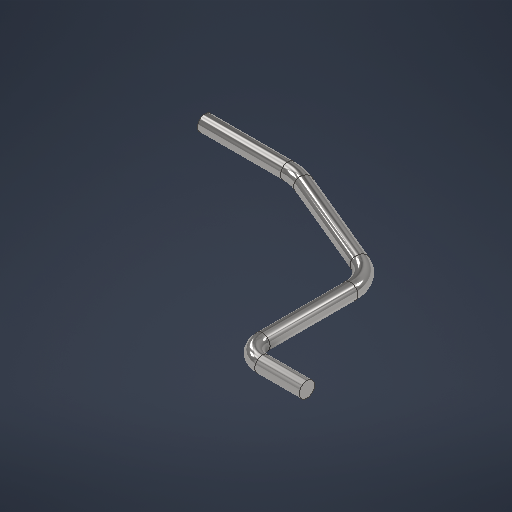
# Autodesk Inventor part: front iron bar
Saved by Autodesk Inventor 2026.1 (Build 301233000, 233)
## iProperties
Created: 2025-12-10
Part Number: front iron bar
Material: Generisch
Document SubType Name: Modeling
Designer: Familie
Density: 1 g/cm^3
Appearance: Stahl - poliert
Author: Familie
Autodesk Inventor part; units mm, degrees
ref_plane "YZ Plane" through (0, 0, 0) normal (1, 0, 0) x (0, 1, 0)
ref_plane "XZ Plane" through (0, 0, 0) normal (0, 1, 0) x (-1, 0, 0)
ref_plane "XY Plane" through (0, 0, 0) normal (0, 0, 1) x (1, 0, 0)
sketch "Skizze1" plane through (0, 0, 0) normal (0, 0, 1) x (1, 0, 0)
  line L0 (0, 0) -> (15, 0)
  arc A0 (20, -1) -> (15, 0) centre (15, -13) ccw
  line L1 (20, -1) -> (45, -11.4167)
  arc A1 (50, -18.9167) -> (45, -11.4167) centre (41.875, -18.9167) ccw
  line L2 (50, -18.9167) -> (50, -41.6467)
  arc A2 (50, -41.6467) -> (55, -46.6467) centre (55, -41.6467) ccw
  line L3 (55, -46.6467) -> (60, -46.6467)
  line L4 (60, -46.6467) -> (66.5, -46.6467)
  line L5 (0, 0) -> (-6.5, 0)
  point P0 (57.5, -46.6467)
  dimension "d0" = 15
  dimension "d1" = 20
  dimension "d2" = 1
  dimension "d3" = 45
  dimension "d4" = 5
  dimension "d5" = 22.73
  dimension "d6" = 5
  dimension "d7" = 5
  dimension "d20" = 46.6467
  dimension "d22" = 6.5
  dimension "d23" = 6.5
  constraints: 12 end point, 6 point on circle, 6 tangent, 4 horizontal, 3 centre point, 1 midpoint, 1 vertical
  measures "d0" distance of L0.start L0.end
  measures "d1" horizontal distance of L1.start L0.start
  measures "d2" vertical distance of L0.end L1.start
  measures "d3" horizontal distance of L0.start L1.end
  measures "d4" horizontal distance of L1.end L2.start
  measures "d5" distance of L2.start L2.end
  measures "d6" horizontal distance of L2.end L3.start
  measures "d7" distance of L3.start L3.end
  measures "d20" distance between parallel lines of L3 L0
  measures "d22" distance of L3.end L4.end
  measures "d23" distance of L0.start L5.end
sketch "Skizze2" plane through (0, 0, 0) normal (1, 0, 0) x (0, 1, 0)
  circle A0 centre (0, 0) radius 2
  dimension "d16" = 4
  constraints: 1 centre point, 1 coincident
  measures "d16" diameter of A0
sweep "Sweeping1" add profiles "Skizze2" path "Skizze1"
equation "\"d22\" = d23"
